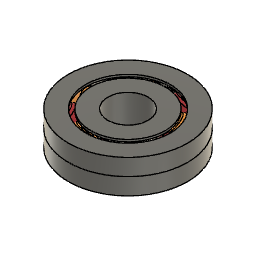
Rodamiento_Giro_V7 (Autodesk Fusion 360 design; units mm, degrees)
Autodesk Fusion 360 part; units mm, degrees
sketch "Top View" plane through (0, 0, 0) normal (0, 0, 1) x (1, 0, 0)
  circle A0 centre (0, 0) radius 13.7176 construction
  ellipse E0 centre (13.7176, 0) end of major axis (19.4451, 0) minor radius 4.05
  line L0 (7.99, 0) -> (19.4451, 0)
  line L1 (13.7176, -4.05) -> (13.7176, 4.05)
  line L2 (0, 0) -> (11.3261, 3.6801) construction
  circle A1 centre (13.7176, 0) radius 5.7276 construction
  line L3 (0, 0) -> (11.3261, 5.2044) construction
  line L4 (11.3261, 5.2044) -> (11.3261, 3.6801) construction
  dimension "d96" = 8.1
  dimension "d97" = 11.4551
  dimension "d98" = 18
  constraint coincident A0.centre L2.start
  constraint coincident A0 E0.centre
  constraint horizontal L0
  constraint coincident E0 L0.start
  constraint coincident E0 L0.end
  constraint coincident E0 L1.start
  constraint coincident E0 L1.end
  constraint coincident A0.centre L0
  constraint coincident E0 L2.end
  constraint concentric E0 A1
  constraint coincident L0.start A1
  constraint coincident A1 L3.end
  constraint tangent A1 L3
  constraint vertical L4
  measures "d97" distance of E0
  measures "d98" angle of L0 L2
sketch "Bearing Section" plane through (0, 0, 0) normal (0, 1, 0) x (1, 0, 0)
  line L0 (7.99, 0) -> (19.4451, 0) construction
  line L1 (7.99, 0) -> (13.7176, 5.7276) construction
  line L2 (13.7176, 5.7276) -> (19.4451, 0) construction
  line L3 (7.99, 0) -> (13.7176, -5.7276) construction
  line L4 (13.7176, -5.7276) -> (19.4451, 0) construction
  line L5 (13.7176, -5.7276) -> (13.7176, 5.7276) construction
  line L6 (10.8538, 2.8638) -> (16.5814, -2.8638) construction
  line L7 (10.8538, -2.8638) -> (16.5814, 2.8638) construction
  line L8 (12.4094, 3.9952) -> (17.7127, -1.3081)
  line L9 (17.7127, -1.3081) -> (18.8441, -0.1768)
  line L10 (18.8441, -0.1768) -> (18.5853, 0.7891)
  line L11 (18.5853, 0.7891) -> (14.5067, 4.8677)
  line L12 (14.5067, 4.8677) -> (13.5408, 5.1265)
  line L13 (13.5408, 5.1265) -> (12.4094, 3.9952)
  line L14 (19.1016, 0) -> (28.2298, 0) construction
  line L15 (14.5176, 5.7266) -> (14.5184, 4.9975)
  line L16 (14.5184, 4.9975) -> (18.8087, 0.7071)
  arc A0 (19.1016, 0) -> (18.8087, 0.7071) centre (18.1016, 0) ccw
  line L17 (14.5184, -4.9975) -> (18.8087, -0.7071)
  line L18 (14.5176, -5.7266) -> (14.5184, -4.9975)
  arc A1 (18.8087, -0.7071) -> (19.1016, 0) centre (18.1016, 0) ccw
  line L19 (12.9176, -5.7266) -> (12.9167, -4.9975)
  line L20 (12.9167, -4.9975) -> (8.6264, -0.7071)
  line L21 (12.9167, 4.9975) -> (8.6264, 0.7071)
  arc A2 (8.6264, 0.7071) -> (8.3335, 0) centre (9.3335, 0) ccw
  arc A3 (8.3335, 0) -> (8.6264, -0.7071) centre (9.3335, 0) ccw
  line L22 (12.9176, 5.7266) -> (12.9167, 4.9975)
  line L23 (12.9176, 5.7266) -> (6.9176, 5.7334)
  line L24 (6.9176, 5.7334) -> (6.9176, 0)
  line L25 (14.5176, 5.7266) -> (20.5176, 5.7334)
  line L26 (20.5176, 5.7334) -> (20.5176, 0)
  line L27 (14.5176, -5.7266) -> (20.5176, -5.7334)
  line L28 (20.5176, -5.7334) -> (20.5176, 0)
  line L29 (11.8457, 0) -> (8.3335, 0)
  line L30 (6.9176, -5.7334) -> (6.9176, 0)
  line L31 (12.9176, -5.7266) -> (6.9176, -5.7334)
  line L32 (19.1016, 0) -> (20.5176, 0)
  dimension "d99" = 0.05
  dimension "d100" = 0.3
  dimension "d101" = 60
  dimension "d102" = 0.5
  dimension "d103" = 1.6
  dimension "d112" = 0.05
  dimension "d113" = 0.8
  dimension "d114" = 1
  dimension "d142" = 6
  dimension "d143" = 6
  constraint coincident L0.start L1.start
  constraint coincident L0.end L2.end
  constraint perpendicular L1 L2
  constraint equal L1 L2
  constraint symmetric L0 L1.start L3.start
  constraint symmetric L0 L1.end L3.end
  constraint symmetric L0 L2.end L4.end
  constraint midpoint L1 L6.start
  constraint midpoint L4 L6.end
  constraint midpoint L3 L7.start
  constraint midpoint L2 L7.end
  constraint symmetric L7 L10.end L11.end
  constraint symmetric L7 L9.end L12.end
  constraint symmetric L7 L8.start L8.end
  constraint parallel L1 L13
  constraint horizontal L14
  constraint tangent L16 A0
  constraint coincident L14 A0.centre
  constraint collinear L0 L14
  constraint parallel L2 L16
  constraint symmetric L0 L14.start A0.start
  constraint symmetric L0 L15.start L18.start
  constraint symmetric L0 L15.end L17.start
  constraint symmetric L0 L16.end L17.end
  constraint symmetric L0 A0 A1
  constraint symmetric L5 L14.start A2.end
  constraint symmetric L5 L15.start L22.start
  constraint symmetric L5 L15.end L21.start
  constraint symmetric L5 L16.end L21.end
  constraint symmetric L5 A0 A2
  constraint symmetric L5 L17.start L19.end
  constraint symmetric L5 L17.end L20.end
  constraint symmetric L5 L18.start L19.start
  constraint symmetric L5 A1 A3
  constraint perpendicular L22 L23
  constraint perpendicular L15 L25
  constraint coincident L14 L26.end
  constraint perpendicular L14 L26
  constraint symmetric L14 L15.start L18.start
  constraint symmetric L14 L25.end L27.end
  constraint symmetric L14 L26.end L28.end
  constraint parallel L24 L26
  constraint symmetric L22.start L29 L19.start
  constraint symmetric L23.end L29 L30.start
  constraint symmetric L24.end L29 L30.end
  constraint parallel L28 L30
  constraint perpendicular L28 L32
  measures "d99" distance of L2 L11
  measures "d100" distance of L1 L13
  measures "d101" angle of L12 L13
  measures "d102" distance of L11 L12.end
  measures "d103" distance of L8.start L12.end
  measures "d112" distance of L2 L16
  measures "d113" distance of L1.end L15
  measures "d114" radius of A0
  measures "d142" distance of L22.start L23.end
  measures "d143" distance of L15.start L25.end
revolve "Revolve1" add sketch "Bearing Section" angle 360 about axis through (10.8538, 0, -2.8638) along (0.707107, 0, 0.707107) contours L8 L9 L10 L11 L12 L13 makes body 1 in component "CilindrosA"
pattern_circular "C-Pattern1" count 5 over 360 about axis through (0, 0, 1.75) along (0, 0, 1) of bodies 1 makes body 2 at (5.5116, 16.3177, -2.1452) makes body 3 at (-13.8159, 10.2843, -2.1452) makes body 4 at (-14.0503, -9.9617, -2.1452) makes body 5 at (5.1323, -16.4409, -2.1452) in component "CilindrosA"
revolve "Revolve1'" add sketch "Bearing Section" angle 360 about axis through (10.8538, 0, -2.8638) along (0.707107, 0, 0.707107) separate body contours L8 L9 L10 L11 L12 L13 makes body 6 in component "CilindrosB"
move_body "Move1" bodies 6 to x (-1, 0, 0) y (0, -1, 0) z (0, 0, 1) at (27.4351, 0, 0) in component "CilindrosB"
move_body "Move2" bodies 6 to x (0.809017, 0.587785, 0) y (-0.587785, 0.809017, 0) z (0, 0, 1) at (0, 0, 0) in component "CilindrosB"
pattern_circular "C-Pattern1'" count 5 over 360 about axis through (0, 0, 1.75) along (0, 0, 1) of bodies 6 makes body 7 at (-3.3456, 9.6514, -2.1452) makes body 8 at (-10.2129, -0.1994, -2.1452) makes body 9 at (-2.9663, -9.7747, -2.1452) makes body 10 at (8.3796, -5.8417, -2.1452) in component "CilindrosB"
revolve "Revolución7" add sketch "Bearing Section" angle 360 about axis through (0, 0, 1.75) along (0, 0, 1) separate body contours L19 L20 L21 A2 A3 L22 L23 L24 L30 L31 makes body 11 in component "Interior"
revolve "Revolución6" add sketch "Bearing Section" angle 360 about axis through (0, 0, 1.75) along (0, 0, 1) separate body contours L17 L18 A1 L27 L28 L32 makes body 12 in component "Exterior"
revolve "Revolución7'" add sketch "Bearing Section" angle 360 about axis through (0, 0, 1.75) along (0, 0, 1) separate body contours L15 L16 A0 L25 L26 L32 makes body 13 in component "Exterior"
sketch "Cut" plane through (0, 0, 0) normal (0, 0, 1) x (1, 0, 0)
  circle A0 centre (0, 0) radius 42.8755
  circle A1 centre (0, 0) radius 40.8755 construction
  line L0 (39.6118, -16.4077) -> (-39.6118, 16.4077)
  line L1 (16.4077, 39.6118) -> (-16.4077, -39.6118)
  point P0 (40.8755, 0)
  dimension "d131" = 2
  dimension "d132" = 54
  constraint coincident A0.centre A1.centre
  constraint coincident P0 A1
  constraint coincident A0 L0.start
  constraint coincident A0 L0.end
  constraint coincident A0 L1.start
  constraint coincident A0 L1.end
  constraint perpendicular L0 L1
  constraint coincident A0.centre L0
  constraint coincident A0.centre L1
  measures "d131" distance of A0 A1
  measures "d132" angle of P0 A0.centre L0.start
component "CilindrosA" placed x (1, 0, 0) y (0, 1, 0) z (0, 0, 1) at (0, 0, 0)
component "CilindrosB" placed x (1, 0, 0) y (0, 1, 0) z (0, 0, 1) at (0, 0, 0)
component "Exterior" placed x (1, 0, 0) y (0, 1, 0) z (0, 0, 1) at (0, 0, 0)
component "Interior" placed x (1, 0, 0) y (0, 1, 0) z (0, 0, 1) at (0, 0, 0)
equation "GapFit = 0.1 mm"
equation "GapSlide = 0.3 mm"
equation "NumRolls = 10"
equation "RollDiameter = 8 mm"
equation "d96 = RollDiameter + GapFit"
equation "d97 = sqrt(2) * d96"
equation "d98 = ( 180 / NumRolls ) * 1 deg"
equation "d99 = GapFit / 2"
equation "d100 = GapSlide"
equation "d105 = NumRolls / 2"
equation "d109 = ( 360 / NumRolls ) * 1 deg"
equation "d110 = NumRolls / 2"
equation "d112 = GapFit / 2"
equation "ScrewDiameter = 1.5 mm"
equation "NumScrews = 12"
equation "d132 = ( 3 * 180 / NumRolls ) * 1 deg"
named bodies: "Interior", "Exterior_Superior", "Exterior_Inferior"
